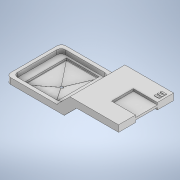
# Autodesk Inventor part: mc_coneholder_3dprint
Saved by Autodesk Inventor 2021 (Build 250183000, 183)
## iProperties
Created: 2021-11-17
Part Number: mc_coneholder_3dprint
Material: Generic
Document SubType Name: Modeling
Designer: mattc
Density: 1 g/cm^3
Appearance: Default
Author: mattc
Autodesk Inventor part; units mm, degrees
ref_plane "YZ Plane" through (0, 0, 0) normal (1, 0, 0) x (0, 1, 0)
ref_plane "XZ Plane" through (0, 0, 0) normal (0, 1, 0) x (-1, 0, 0)
ref_plane "XY Plane" through (0, 0, 0) normal (0, 0, 1) x (1, 0, 0)
sketch "cone top" plane through (0, 0, 0) normal (0, 1, 0) x (-1, 0, 0)
  line L0 (-7.5, 10) -> (7.5, 10)
  line L1 (7.5, 10) -> (7.5, -10)
  line L2 (7.5, -10) -> (-7.5, -10)
  line L3 (-7.5, -10) -> (-7.5, 10)
  line L4 (-7.5, 10) -> (7.5, -10) construction
  line L5 (7.5, 10) -> (-7.5, -10) construction
  point P0 (0, 0)
  dimension "d0" = 15
  dimension "d1" = 20
  constraints: 12 end point, 2 midpoint, 2 parallel, 1 horizontal, 1 perpendicular
  measures "d0" distance of L1.end L2.end
  measures "d1" distance of L0.end L1.end
ref_plane "Work Plane2" through (0, -2.25, 0) normal (0, 1, 0) x (-1, 0, 0)
sketch "fly slot" plane through (0, -2.25, 0) normal (0, 1, 0) x (-1, 0, 0)
  spline S0 degree 4 poles (0.396397, -0.000152) (0.398365, -0.036035) (0.401106, -0.11328) (0.340029, -0.23723) (0.205161, -0.447077) (-0.39841, -0.389238) (-0.771706, -0.382709) (-1.027545, -0.147082) (-1.226778, -0.000152) knots 0 0 0 0 0 0.0981587 0.21107942 0.37180814 0.54451889 1 1 1 1 1
  line L0 (0.396397, -0.000152) -> (-1.226778, -0.000152)
  spline S1 degree 4 poles (0.396397, -0.000152) (0.394448, 0.035396) (0.388793, 0.111758) (0.357394, 0.238637) (0.192883, 0.445563) (-0.385091, 0.390246) (-0.78204, 0.381387) (-1.021951, 0.147329) (-1.226778, -0.000152) knots 0 0 0 0 0 0.0981587 0.21107942 0.37180814 0.54451889 1 1 1 1 1
  point P0 (0.36514, -0.178249)
  point P1 (0.218618, -0.361523)
  point P2 (-0.589473, -0.361523)
  point P3 (-0.909157, -0.229309)
  point P4 (-0.169887, -0.412583)
  point P5 (0.36514, 0.177945)
  point P6 (0.218618, 0.361218)
  point P7 (-0.589473, 0.361218)
  point P8 (-0.909157, 0.229005)
  point P9 (-0.169887, 0.412279)
  constraints: 5 symmetric about line, 2 end point, 14 other
sketch "Sketch6" plane through (0, -2.25, 0) normal (0, 1, 0) x (-1, 0, 0)
  line L0 (-0.01655, -0.031342) -> (0.01655, -0.031342)
  line L1 (0.01655, -0.031342) -> (0.01655, 0.031342)
  line L2 (0.01655, 0.031342) -> (-0.01655, 0.031342)
  line L3 (-0.01655, 0.031342) -> (-0.01655, -0.031342)
  line L4 (-0.01655, -0.031342) -> (0.01655, 0.031342) construction
  line L5 (0.01655, -0.031342) -> (-0.01655, 0.031342) construction
  point P0 (0, 0)
  constraints: 12 end point, 2 midpoint, 2 parallel, 1 horizontal, 1 perpendicular
loft "Loft3" add profiles "cone top", "Sketch6"
shell "Shell1" thickness 0.08 removed faces 1 at (2.5, 0, 3.333333)
extrude "Extrusion4" cut sketch "fly slot" along normal blind 10
ref_plane "Work Plane3" through (-7.5, 0, 10) normal (0, 1, 0) x (1, 0, 0)
sketch "Sketch7" plane through (-7.5, 0, 10) normal (0, 1, 0) x (1, 0, 0)
  line L0 (20, 22.65) -> (-5, 22.65)
  line L1 (-5, 22.65) -> (-5, -2.65)
  line L2 (-5, -2.65) -> (20, -2.65)
  line L3 (20, -2.65) -> (20, 22.65)
  line L4 (20, 22.65) -> (-5, -2.65) construction
  line L5 (-5, 22.65) -> (20, -2.65) construction
  line L6 (15, 0) -> (7.795496, 9.597074)
  line L7 (0, 20) -> (15, 20)
  line L8 (15, 20) -> (15, 0)
  line L9 (15, 0) -> (0, 0)
  line L10 (0, 0) -> (0, 20)
  line L11 (0, 20) -> (15, 0) construction
  line L12 (15, 20) -> (0, 0) construction
  point P0 (7.5, 10)
  dimension "d32" = 25
  dimension "d33" = 25.3
  constraints: 24 end point, 4 midpoint, 4 parallel, 2 horizontal, 2 perpendicular
  measures "d32" distance of L2.end L1.end
  measures "d33" distance of L1.end L0.end
extrude "Extrusion5" add sketch "Sketch7" along normal blind 0.75
sketch "Sketch8" plane through (-7.5, 0.75, 10) normal (0, 1, 0) x (1, 0, 0)
  line L0 (-5, -2.65) -> (20, -2.65) projected
  line L1 (-5, 22.65) -> (20, 22.65)
  line L2 (20, 22.65) -> (20, -2.65)
  line L3 (20, -2.65) -> (-5, -2.65)
  line L4 (-5, -2.65) -> (-5, 22.65)
  line L5 (-5, 22.65) -> (20, -2.65) construction
  line L6 (20, 22.65) -> (-5, -2.65) construction
  line L7 (-3.5, 21) -> (18.5, 21)
  line L8 (18.5, 21) -> (18.5, -1)
  line L9 (18.5, -1) -> (-3.5, -1)
  line L10 (-3.5, -1) -> (-3.5, 21)
  line L11 (-3.5, 21) -> (18.5, -1) construction
  line L12 (18.5, 21) -> (-3.5, -1) construction
  point P0 (7.5, 10)
  dimension "d36" = 22
  dimension "d37" = 22
  constraints: 24 end point, 4 midpoint, 4 parallel, 2 horizontal, 2 perpendicular
  measures "d36" distance of L8.end L9.end
  measures "d37" distance of L7.end L8.end
extrude "Extrusion6" add sketch "Sketch8" along normal blind 2
move faces "Move1" translate (1.588, 0, 0) faces at (12.5, 1.833333, -4.216667)
sketch "Sketch9" plane through (-7.5, 2.75, 10) normal (0, 1, 0) x (1, 0, 0)
  line L0 (-5, -2.65) -> (21.588, -2.65)
  line L1 (21.588, 22.65) -> (18.500223, 22.65)
  line L2 (18.500223, 22.65) -> (18.500223, -2.65)
  line L3 (18.500223, -2.65) -> (21.588, -2.65)
  line L4 (21.588, -2.65) -> (21.588, 22.65)
  point P0 (7.5, 10)
  point P1 (21.588, -2.65)
  constraints: 8 end point, 2 parallel, 1 horizontal, 1 perpendicular, 1 point on line
extrude "Extrusion7" add sketch "Sketch9" along normal blind 6
sketch "Sketch10" plane through (14.088, 0, 12.65) normal (1, 0, 0) x (0, 0, -1)
  line L0 (0, 0) -> (0, 8.75) projected
  line L1 (25.3, 0) -> (25.3, 8.75) projected
  line L2 (0, 8.75) -> (25.3, 8.75)
  line L3 (25.3, 8.75) -> (25.3, 5.75)
  line L4 (25.3, 5.75) -> (0, 5.75)
  line L5 (0, 5.75) -> (0, 8.75)
  point P0 (12.65, 0)
  point P1 (0, 5.75)
  dimension "d45" = 3
  constraints: 8 end point, 2 parallel, 1 horizontal, 1 perpendicular, 1 point on line
  measures "d45" distance of L2.end L3.end
extrude "Extrusion8" add sketch "Sketch10" along normal blind 25
sketch "Sketch11" plane through (14.088, 5.75, -12.65) normal (0, -1, 0) x (1, 0, 0)
  line L0 (25, 0) -> (25, 25.3) projected
  line L1 (25, 7.5) -> (14, 7.5)
  line L2 (14, 7.5) -> (14, 17.5)
  line L3 (14, 17.5) -> (25, 17.5)
  line L4 (25, 17.5) -> (25, 7.5)
  point P0 (-14.088, 12.65)
  dimension "d48" = 11
  dimension "d49" = 10
  constraints: 8 end point, 2 parallel, 1 horizontal, 1 perpendicular, 1 point on line
  measures "d48" distance of L2.end L3.end
  measures "d49" distance of L1.end L2.end
extrude "Extrusion9" cut sketch "Sketch11" against normal blind 1
sketch "Sketch12" plane through (-7.5, 8.75, 10) normal (0, 1, 0) x (1, 0, 0)
  line L0 (46.588, -2.65) -> (46.588, 5.15)
  line L1 (46.588, 0.002536) -> (17.245955, 0.002536)
  line L2 (17.245955, 0.002536) -> (17.245955, 3.002536)
  line L3 (17.245955, 3.002536) -> (46.588, 3.002536)
  line L4 (46.588, 3.002536) -> (46.588, 0.002536)
  point P0 (7.5, 10)
  point P1 (46.588, 3.002536)
  dimension "d52" = 3
  constraints: 8 end point, 2 parallel, 1 horizontal, 1 perpendicular, 1 point on line
  measures "d52" distance of L1.end L2.end
extrude "Extrusion10" [suppressed]
chamfer "Chamfer1" distance 5.7 angle 45 1 edges at (14.088, 5.75, 0)
chamfer "Chamfer2" distance 5.7 angle 45 1 edges at (11.0002, 8.75, 0)
fillet "Fillet2" radius 2 4 edges at (11, 1.75, -11) (11, 1.75, 11) (-11, 1.75, -11) (-11, 1.75, 11)
sketch "Sketch13" plane through (-7.5, 8.75, 10) normal (0, 1, 0) x (1, 0, 0)
  line L0 (46.588, 15.15) -> (35.588, 15.15) projected
  line L1 (35.588, 5.15) -> (46.588, 5.15) projected
  line L2 (35.588, 15.15) -> (46.588, 15.15)
  line L3 (46.588, 15.15) -> (46.588, 5.15)
  line L4 (46.588, 5.15) -> (35.588, 5.15)
  line L5 (35.588, 5.15) -> (35.588, 15.15)
  point P0 (7.5, 10)
  constraints: 8 end point, 2 parallel, 1 horizontal, 1 perpendicular
extrude "Extrusion11" cut sketch "Sketch13" against normal blind 1
fillet "Fillet3" radius 2 2 edges at (-12.5, 1.375, -12.65) (-12.5, 1.375, 12.65)
sketch "Sketch14" plane through (-7.5, 8.75, 10) normal (0, 1, 0) x (1, 0, 0)
  line L0 (45.602193, 20.774988) -> (45.602193, 17.255215) construction
  line L1 (45.602193, 17.255215) -> (43.250738, 17.255215) construction
  line L2 (43.250738, 17.255215) -> (43.250738, 20.774988) construction
  line L3 (43.250738, 20.774988) -> (45.602193, 20.774988) construction
  line L4 (43.239308, 17.754648) -> (44.388619, 17.754648)
  spline S0 degree 2 poles (44.388619, 17.754648) (44.559162, 17.754648) (44.791496, 17.767006) (44.865645, 17.796666) knots 0 0 0 1 2 2 2
  spline S1 degree 2 poles (44.865645, 17.796666) (44.939794, 17.828797) (45.006529, 17.957322) (45.006529, 18.073489) knots 0 0 0 1 2 2 2
  spline S2 degree 2 poles (45.006529, 18.073489) (45.006529, 18.155053) (44.934851, 18.313238) (44.868117, 18.40716) knots 0 0 0 1 2 2 2
  line L5 (44.868117, 18.40716) -> (43.239308, 18.40716)
  line L6 (43.239308, 18.40716) -> (43.239308, 19.128878)
  line L7 (43.239308, 19.128878) -> (44.388619, 19.128878)
  spline S3 degree 2 poles (44.388619, 19.128878) (44.556691, 19.128878) (44.791496, 19.143708) (44.865645, 19.173368) knots 0 0 0 1 2 2 2
  spline S4 degree 2 poles (44.865645, 19.173368) (44.939794, 19.205499) (45.006529, 19.334024) (45.006529, 19.450191) knots 0 0 0 1 2 2 2
  spline S5 degree 2 poles (45.006529, 19.450191) (45.006529, 19.536698) (44.924965, 19.707241) (44.868117, 19.786334) knots 0 0 0 1 2 2 2
  line L8 (44.868117, 19.786334) -> (43.239308, 19.786334)
  line L9 (43.239308, 19.786334) -> (43.239308, 20.503108)
  line L10 (43.239308, 20.503108) -> (45.540402, 20.503108)
  line L11 (45.540402, 20.503108) -> (45.540402, 19.786334)
  line L12 (45.540402, 19.786334) -> (45.285824, 19.786334)
  spline S6 degree 2 poles (45.285824, 19.786334) (45.434122, 19.610847) (45.602193, 19.296949) (45.602193, 19.10169) knots 0 0 0 1 2 2 2
  spline S7 degree 2 poles (45.602193, 19.10169) (45.602193, 18.891601) (45.401991, 18.570288) (45.201788, 18.486253) knots 0 0 0 1 2 2 2
  spline S8 degree 2 poles (45.201788, 18.486253) (45.394576, 18.281107) (45.602193, 17.915304) (45.602193, 17.72746) knots 0 0 0 1 2 2 2
  spline S9 degree 2 poles (45.602193, 17.72746) (45.602193, 17.566804) (45.500856, 17.312225) (45.397047, 17.225718) knots 0 0 0 1 2 2 2
  spline S10 degree 2 poles (45.397047, 17.225718) (45.285824, 17.129324) (44.981812, 17.03293) (44.73712, 17.03293) knots 0 0 0 1 2 2 2
  line L13 (44.73712, 17.03293) -> (43.239308, 17.03293)
  line L14 (43.239308, 17.03293) -> (43.239308, 17.754648)
  point P0 (7.5, 10)
  constraints: 2 other
emboss "Emboss1" sketch "Sketch14" operation add depth 0.2 direction (0, -1, 0)
body "Solid4"
